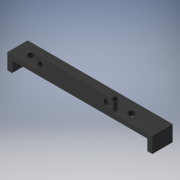
# Autodesk Inventor part: PSUMount
Saved by Autodesk Inventor 2019.1 (Build 231200000, 200)
## iProperties
Created: 2019-10-07
Part Number: PSUMount
Material: Generic
Document SubType Name: Modeling
Designer: Computus
Density: 1 g/cm^3
Appearance: Default
Author: Computus
Autodesk Inventor part; units mm, degrees
ref_plane "YZ Plane" through (0, 0, 0) normal (1, 0, 0) x (0, 1, 0)
ref_plane "XZ Plane" through (0, 0, 0) normal (0, 1, 0) x (-1, 0, 0)
ref_plane "XY Plane" through (0, 0, 0) normal (0, 0, 1) x (1, 0, 0)
sketch "Sketch1" plane through (0, 0, 0) normal (0, 1, 0) x (-1, 0, 0)
  line L0 (0, 0) -> (93, 0)
  line L1 (93, 0) -> (93, -13)
  line L2 (93, -13) -> (0, -13)
  line L3 (0, -13) -> (0, 0)
  circle A0 centre (83.5, -6) radius 2.4
  circle A1 centre (19, -6) radius 2.4
  dimension "d0" = 93
  dimension "d1" = 13
  dimension "d2" = 4.8
  dimension "d3" = 4.8
  dimension "d4" = 6
  dimension "d5" = 6
  dimension "d6" = 19
  dimension "d7" = 9.5
  constraints: 8 end point, 2 centre point, 2 parallel, 1 horizontal, 1 perpendicular
  measures "d0" distance of L1.end L2.end
  measures "d1" distance of L0.end L1.end
  measures "d2" diameter of A0
  measures "d3" diameter of A1
  measures "d4" distance from line of A0.centre L0
  measures "d5" distance from line of A1.centre L0
  measures "d6" distance from line of L3 A1.centre
  measures "d7" distance from line of L1 A0.centre
extrude "Extrusion1" add sketch "Sketch1" along normal blind 3
sketch "Sketch2" plane through (0, 3, 0) normal (0, 1, 0) x (1, 0, 0)
  line L0 (-93, 0) -> (0, 0) projected
  line L1 (0, 13) -> (-93, 13) projected
  line L2 (0, 0) -> (-3, 0)
  line L3 (-3, 0) -> (-3, 13)
  line L4 (-3, 13) -> (0, 13)
  line L5 (0, 13) -> (0, 0)
  line L6 (-93, 0) -> (-90, 0)
  line L7 (-90, 0) -> (-90, 13)
  line L8 (-90, 13) -> (-93, 13)
  line L9 (-93, 13) -> (-93, 0)
  dimension "d10" = 3
  dimension "d11" = 3
  constraints: 16 end point, 4 parallel, 2 horizontal, 2 perpendicular, 2 point on line
  measures "d10" distance of L3.end L4.end
  measures "d11" distance of L8.end L7.end
extrude "Extrusion2" add sketch "Sketch2" against normal blind 10 contours L9 L1 L7 L0 | L3 L1 L5 L0
sketch "Sketch3" plane through (0, 3, 0) normal (0, 1, 0) x (1, 0, 0)
  line L0 (-3, 0) -> (-90, 0) projected
  line L1 (-75.0955, 0) -> (-25.0955, 0)
  line L2 (-25.0955, 0) -> (-25.0955, 3)
  line L3 (-25.0955, 3) -> (-75.0955, 3)
  line L4 (-75.0955, 3) -> (-75.0955, 0)
  point P0 (0, 0)
  dimension "d14" = 50
  dimension "d15" = 3
  constraints: 8 end point, 2 parallel, 1 horizontal, 1 perpendicular, 1 point on line
  measures "d14" distance of L3.end L2.end
  measures "d15" distance of L2.end L1.end
extrude "Extrusion3" add sketch "Sketch3" along normal blind 8
fillet "Fillet1" radius 2 2 edges at (-25.0955, 11, -1.5) (-75.0955, 11, -1.5)
sketch "Sketch4" plane through (-25.0955, 3, -3) normal (0, 0, -1) x (-1, 0, 0)
  circle A0 centre (46, 4) radius 2.4
  circle A1 centre (4, 4) radius 2.4
  line L0 (2, 8) -> (48, 8) projected
  line L1 (0, 0) -> (0, 6) projected
  line L2 (50, 0) -> (50, 6) projected
  point P0 (-25.0955, -3)
  dimension "d19" = 4.8
  dimension "d20" = 4.8
  dimension "d21" = 4
  dimension "d22" = 4
  dimension "d23" = 4
  dimension "d24" = 4
  constraints: 2 centre point
  measures "d19" diameter of A0
  measures "d20" diameter of A1
  measures "d21" distance from line of L0 A0.centre
  measures "d22" distance from line of L0 A1.centre
  measures "d23" distance from line of L1 A1.centre
  measures "d24" distance from line of L2 A0.centre
extrude "Extrusion4" cut sketch "Sketch4" against normal blind 8
fillet "Fillet2" radius 1 2 edges at (-68.6955, 7, -3) (-26.6955, 7, -3)
body "Solid1"
